Autodesk Inventor part; units mm, degrees
(part 2 of 2)
  spline S324 degree 2 poles (-2.8831, -28.3375) (-2.6289, -28.3375) (-2.4265, -28.3012) (-2.2631, -28.1845) (-2.2009, -28.0807) knots 0 0 0 1 2 3 3 3
  line L148 (-2.2009, -28.0807) -> (-2.1152, -28.0807)
  line L149 (-1.6639, -28.7551) -> (-1.6639, -28.6695)
  spline S325 degree 2 poles (-1.6639, -28.6695) (-1.3578, -28.6644) (-0.8338, -28.392) (-0.3436, -27.7072) (-0.245, -27.2973) knots 0 0 0 1 2 3 3 3
  spline S326 degree 2 poles (-0.245, -27.2973) (-0.6134, -27.5334) (-0.9117, -27.5334) knots 0 0 0 1 1 1
  spline S327 degree 2 poles (-0.9117, -27.5334) (-1.2489, -27.5334) (-1.7262, -27.0172) (-1.7262, -26.5866) knots 0 0 0 1 2 2 2
  spline S328 degree 2 poles (-1.7262, -26.5866) (-1.7262, -26.1716) (-1.4875, -25.8447) knots 0 0 0 1 1 1
  spline S329 degree 2 poles (-1.4875, -25.8447) (-1.1996, -25.4504) (-0.7353, -25.4504) knots 0 0 0 1 1 1
  spline S330 degree 2 poles (-0.7353, -25.4504) (-0.3436, -25.4504) (-0.0634, -25.7747) knots 0 0 0 1 1 1
  spline S331 degree 2 poles (-0.0634, -25.7747) (0.279, -26.1742) (0.279, -26.7604) knots 0 0 0 1 1 1
  spline S332 degree 2 poles (0.279, -26.7604) (0.279, -27.2896) (-0.2424, -28.2052) (-0.7067, -28.5061) knots 0 0 0 1 2 2 2
  spline S333 degree 2 poles (-0.7067, -28.5061) (-1.0855, -28.7551) (-1.529, -28.7551) knots 0 0 0 1 1 1
  line L150 (-1.529, -28.7551) -> (-1.6639, -28.7551)
  spline S334 degree 2 poles (-0.2087, -27.1235) (-0.1672, -26.8201) (-0.1672, -26.6385) knots 0 0 0 1 1 1
  spline S335 degree 2 poles (-0.1672, -26.6385) (-0.1672, -26.4102) (-0.3228, -25.8836) (-0.6056, -25.6035) (-0.7871, -25.6035) knots 0 0 0 1 2 3 3 3
  spline S336 degree 2 poles (-0.7871, -25.6035) (-0.9947, -25.6035) (-1.3085, -25.977) (-1.3085, -26.348) knots 0 0 0 1 2 2 2
  spline S337 degree 2 poles (-1.3085, -26.348) (-1.3085, -26.8408) (-1.101, -27.1184) knots 0 0 0 1 1 1
  spline S338 degree 2 poles (-1.101, -27.1184) (-0.948, -27.3207) (-0.7249, -27.3207) knots 0 0 0 1 1 1
  spline S339 degree 2 poles (-0.7249, -27.3207) (-0.6159, -27.3207) (-0.3202, -27.2169) (-0.2087, -27.1235) knots 0 0 0 1 2 2 2
  line L151 (2.5668, -25.5153) -> (2.3853, -25.9122)
  line L152 (2.3853, -25.9122) -> (1.4307, -25.9122)
  line L153 (1.4307, -25.9122) -> (1.2206, -26.3376)
  spline S340 degree 2 poles (1.2206, -26.3376) (1.8405, -26.4284) (2.2037, -26.7993) knots 0 0 0 1 1 1
  spline S341 degree 2 poles (2.2037, -26.7993) (2.515, -27.1184) (2.515, -27.549) knots 0 0 0 1 1 1
  spline S342 degree 2 poles (2.515, -27.549) (2.515, -27.798) (2.31, -28.226) (2.0014, -28.5243) (1.812, -28.6151) knots 0 0 0 1 2 3 3 3
  spline S343 degree 2 poles (1.812, -28.6151) (1.5422, -28.7448) (1.2595, -28.7448) knots 0 0 0 1 1 1
  spline S344 degree 2 poles (1.2595, -28.7448) (0.9716, -28.7448) (0.7122, -28.5502) (0.7122, -28.4335) knots 0 0 0 1 2 2 2
  spline S345 degree 2 poles (0.7122, -28.4335) (0.7122, -28.3686) (0.8185, -28.2675) (0.9015, -28.2675) knots 0 0 0 1 2 2 2
  spline S346 degree 2 poles (0.9015, -28.2675) (0.9612, -28.2675) (1.0546, -28.3064) (1.1635, -28.3842) knots 0 0 0 1 2 2 2
  spline S347 degree 2 poles (1.1635, -28.3842) (1.3399, -28.5035) (1.5215, -28.5061) knots 0 0 0 1 1 1
  spline S348 degree 2 poles (1.5215, -28.5061) (1.7938, -28.5061) (2.2115, -28.0911) (2.2115, -27.7928) knots 0 0 0 1 2 2 2
  spline S349 degree 2 poles (2.2115, -27.7928) (2.2115, -27.5049) (1.8405, -27.0042) (1.5137, -26.8693) knots 0 0 0 1 2 2 2
  spline S350 degree 2 poles (1.5137, -26.8693) (1.2595, -26.763) (0.8185, -26.7474) knots 0 0 0 1 1 1
  line L154 (0.8185, -26.7474) -> (1.4281, -25.5153)
  line L155 (1.4281, -25.5153) -> (2.5668, -25.5153)
  spline S351 degree 2 poles (3.0571, -27.121) (3.0571, -26.5788) (3.3839, -25.7954) (3.6563, -25.6035) knots 0 0 0 1 2 2 2
  spline S352 degree 2 poles (3.6563, -25.6035) (3.8664, -25.4504) (4.0921, -25.4504) knots 0 0 0 1 1 1
  spline S353 degree 2 poles (4.0921, -25.4504) (4.4578, -25.4504) (4.7484, -25.8214) knots 0 0 0 1 1 1
  spline S354 degree 2 poles (4.7484, -25.8214) (5.1115, -26.2831) (5.1115, -27.0717) knots 0 0 0 1 1 1
  spline S355 degree 2 poles (5.1115, -27.0717) (5.1115, -27.6242) (4.7925, -28.3972) (4.2996, -28.7448) (4.0687, -28.7448) knots 0 0 0 1 2 3 3 3
  spline S356 degree 2 poles (4.0687, -28.7448) (3.6148, -28.7448) (3.3113, -28.2078) knots 0 0 0 1 1 1
  spline S357 degree 2 poles (3.3113, -28.2078) (3.0571, -27.7565) (3.0571, -27.121) knots 0 0 0 1 1 1
  spline S358 degree 2 poles (3.5162, -27.1806) (3.5162, -27.8343) (3.677, -28.2493) knots 0 0 0 1 1 1
  spline S359 degree 2 poles (3.677, -28.2493) (3.8119, -28.5969) (4.0765, -28.5969) knots 0 0 0 1 1 1
  spline S360 degree 2 poles (4.0765, -28.5969) (4.2036, -28.5969) (4.4734, -28.3712) (4.5434, -28.1041) knots 0 0 0 1 2 2 2
  spline S361 degree 2 poles (4.5434, -28.1041) (4.6524, -27.702) (4.6524, -26.9705) knots 0 0 0 1 1 1
  spline S362 degree 2 poles (4.6524, -26.9705) (4.6524, -26.4258) (4.5408, -26.0652) knots 0 0 0 1 1 1
  spline S363 degree 2 poles (4.5408, -26.0652) (4.4552, -25.7954) (4.3229, -25.6839) knots 0 0 0 1 1 1
  spline S364 degree 2 poles (4.3229, -25.6839) (4.227, -25.6061) (4.0895, -25.6061) knots 0 0 0 1 1 1
  spline S365 degree 2 poles (4.0895, -25.6061) (3.9313, -25.6061) (3.8067, -25.7488) knots 0 0 0 1 1 1
  spline S366 degree 2 poles (3.8067, -25.7488) (3.6381, -25.9433) (3.5162, -26.776) (3.5162, -27.1806) knots 0 0 0 1 2 2 2
  spline S367 degree 2 poles (5.4565, -27.121) (5.4565, -26.5788) (5.7833, -25.7954) (6.0557, -25.6035) knots 0 0 0 1 2 2 2
  spline S368 degree 2 poles (6.0557, -25.6035) (6.2658, -25.4504) (6.4915, -25.4504) knots 0 0 0 1 1 1
  spline S369 degree 2 poles (6.4915, -25.4504) (6.8572, -25.4504) (7.1478, -25.8214) knots 0 0 0 1 1 1
  spline S370 degree 2 poles (7.1478, -25.8214) (7.5109, -26.2831) (7.5109, -27.0717) knots 0 0 0 1 1 1
  spline S371 degree 2 poles (7.5109, -27.0717) (7.5109, -27.6242) (7.1919, -28.3972) (6.699, -28.7448) (6.4681, -28.7448) knots 0 0 0 1 2 3 3 3
  spline S372 degree 2 poles (6.4681, -28.7448) (6.0142, -28.7448) (5.7107, -28.2078) knots 0 0 0 1 1 1
  spline S373 degree 2 poles (5.7107, -28.2078) (5.4565, -27.7565) (5.4565, -27.121) knots 0 0 0 1 1 1
  spline S374 degree 2 poles (5.9156, -27.1806) (5.9156, -27.8343) (6.0765, -28.2493) knots 0 0 0 1 1 1
  spline S375 degree 2 poles (6.0765, -28.2493) (6.2113, -28.5969) (6.4759, -28.5969) knots 0 0 0 1 1 1
  spline S376 degree 2 poles (6.4759, -28.5969) (6.603, -28.5969) (6.8728, -28.3712) (6.9428, -28.1041) knots 0 0 0 1 2 2 2
  spline S377 degree 2 poles (6.9428, -28.1041) (7.0518, -27.702) (7.0518, -26.9705) knots 0 0 0 1 1 1
  spline S378 degree 2 poles (7.0518, -26.9705) (7.0518, -26.4258) (6.9402, -26.0652) knots 0 0 0 1 1 1
  spline S379 degree 2 poles (6.9402, -26.0652) (6.8546, -25.7954) (6.7224, -25.6839) knots 0 0 0 1 1 1
  spline S380 degree 2 poles (6.7224, -25.6839) (6.6264, -25.6061) (6.4889, -25.6061) knots 0 0 0 1 1 1
  spline S381 degree 2 poles (6.4889, -25.6061) (6.3307, -25.6061) (6.2062, -25.7488) knots 0 0 0 1 1 1
  spline S382 degree 2 poles (6.2062, -25.7488) (6.0375, -25.9433) (5.9156, -26.776) (5.9156, -27.1806) knots 0 0 0 1 2 2 2
  line L156 (8.2424, -25.8266) -> (9.0154, -25.4504)
  line L157 (9.0154, -25.4504) -> (9.0932, -25.4504)
  line L158 (9.0932, -25.4504) -> (9.0932, -28.13)
  spline S383 degree 2 poles (9.0932, -28.13) (9.0932, -28.3972) (9.1373, -28.5295) (9.2774, -28.5995) (9.4927, -28.6047) knots 0 0 0 1 2 3 3 3
  line L159 (9.4927, -28.6047) -> (9.4927, -28.6903)
  line L160 (9.4927, -28.6903) -> (8.2995, -28.6903)
  line L161 (8.2995, -28.6903) -> (8.2995, -28.6047)
  spline S384 degree 2 poles (8.2995, -28.6047) (8.5252, -28.5995) (8.6548, -28.5321) (8.7067, -28.4179) (8.7067, -28.13) knots 0 0 0 1 2 3 3 3
  line L162 (8.7067, -28.13) -> (8.7067, -26.418)
  spline S385 degree 2 poles (8.7067, -26.418) (8.7067, -26.0704) (8.6834, -25.9718) knots 0 0 0 1 1 1
  spline S386 degree 2 poles (8.6834, -25.9718) (8.6678, -25.8966) (8.5796, -25.8266) (8.52, -25.8266) knots 0 0 0 1 2 2 2
  spline S387 degree 2 poles (8.52, -25.8266) (8.4318, -25.8266) (8.2787, -25.8992) knots 0 0 0 1 1 1
  line L163 (8.2787, -25.8992) -> (8.2424, -25.8266)
  line L164 (-12.1098, -33.1024) -> (-12.3328, -33.712)
  line L165 (-12.3328, -33.712) -> (-14.2057, -33.712)
  line L166 (-14.2057, -33.712) -> (-14.2057, -33.6264)
  spline S388 degree 2 poles (-14.2057, -33.6264) (-13.3782, -32.8716) (-12.7038, -31.917) (-12.7038, -31.5201) knots 0 0 0 1 2 2 2
  spline S389 degree 2 poles (-12.7038, -31.5201) (-12.7038, -31.2192) (-13.0747, -30.8301) (-13.3315, -30.8301) knots 0 0 0 1 2 2 2
  spline S390 degree 2 poles (-13.3315, -30.8301) (-13.5676, -30.8301) (-13.9385, -31.1051) (-14.0293, -31.3697) knots 0 0 0 1 2 2 2
  line L167 (-14.0293, -31.3697) -> (-14.1149, -31.3697)
  spline S391 degree 2 poles (-14.1149, -31.3697) (-14.0552, -30.9365) (-13.5727, -30.4722) (-13.2096, -30.4722) knots 0 0 0 1 2 2 2
  spline S392 degree 2 poles (-13.2096, -30.4722) (-12.8231, -30.4722) (-12.3043, -30.9676) (-12.3043, -31.3048) knots 0 0 0 1 2 2 2
  spline S393 degree 2 poles (-12.3043, -31.3048) (-12.3043, -31.5461) (-12.4158, -31.7873) knots 0 0 0 1 1 1
  spline S394 degree 2 poles (-12.4158, -31.7873) (-12.5896, -32.166) (-12.9787, -32.5914) knots 0 0 0 1 1 1
  spline S395 degree 2 poles (-12.9787, -32.5914) (-13.5624, -33.2269) (-13.7076, -33.3592) knots 0 0 0 1 1 1
  line L168 (-13.7076, -33.3592) -> (-12.8776, -33.3592)
  spline S396 degree 2 poles (-12.8776, -33.3592) (-12.6234, -33.3592) (-12.421, -33.3229) (-12.2576, -33.2062) (-12.1954, -33.1024) knots 0 0 0 1 2 3 3 3
  line L169 (-12.1954, -33.1024) -> (-12.1098, -33.1024)
  spline S397 degree 2 poles (-10.9892, -32.1115) (-11.3653, -31.8029) (-11.5832, -31.4293) (-11.5832, -31.227) knots 0 0 0 1 2 2 2
  spline S398 degree 2 poles (-11.5832, -31.227) (-11.5832, -30.9183) (-11.1059, -30.4722) (-10.709, -30.4722) knots 0 0 0 1 2 2 2
  spline S399 degree 2 poles (-10.709, -30.4722) (-10.3251, -30.4722) (-9.8556, -30.8872) (-9.8556, -31.1544) knots 0 0 0 1 2 2 2
  spline S400 degree 2 poles (-9.8556, -31.1544) (-9.8556, -31.3334) (-10.1098, -31.7017) (-10.5093, -31.9533) knots 0 0 0 1 2 2 2
  spline S401 degree 2 poles (-10.5093, -31.9533) (-10.0968, -32.2698) (-9.9646, -32.4539) knots 0 0 0 1 1 1
  spline S402 degree 2 poles (-9.9646, -32.4539) (-9.7856, -32.6926) (-9.7856, -32.9572) knots 0 0 0 1 1 1
  spline S403 degree 2 poles (-9.7856, -32.9572) (-9.7856, -33.2918) (-10.2966, -33.7665) (-10.7116, -33.7665) knots 0 0 0 1 2 2 2
  spline S404 degree 2 poles (-10.7116, -33.7665) (-11.1656, -33.7665) (-11.4172, -33.4837) knots 0 0 0 1 1 1
  spline S405 degree 2 poles (-11.4172, -33.4837) (-11.6195, -33.2555) (-11.6195, -32.9857) knots 0 0 0 1 1 1
  spline S406 degree 2 poles (-11.6195, -32.9857) (-11.6195, -32.7756) (-11.3368, -32.3632) (-10.9892, -32.1115) knots 0 0 0 1 2 2 2
  spline S407 degree 2 poles (-10.8776, -32.1997) (-11.0748, -32.3632) (-11.2615, -32.7497) (-11.2615, -32.9753) knots 0 0 0 1 2 2 2
  spline S408 degree 2 poles (-11.2615, -32.9753) (-11.2615, -33.2762) (-10.9295, -33.6394) (-10.6753, -33.6394) knots 0 0 0 1 2 2 2
  spline S409 degree 2 poles (-10.6753, -33.6394) (-10.4211, -33.6394) (-10.115, -33.354) (-10.115, -33.1491) knots 0 0 0 1 2 2 2
  spline S410 degree 2 poles (-10.115, -33.1491) (-10.115, -32.9831) (-10.2032, -32.8482) knots 0 0 0 1 1 1
  spline S411 degree 2 poles (-10.2032, -32.8482) (-10.3718, -32.6018) (-10.8776, -32.1997) knots 0 0 0 1 1 1
  spline S412 degree 2 poles (-10.6208, -31.8599) (-10.3381, -31.6083) (-10.1876, -31.3152) (-10.1876, -31.131) knots 0 0 0 1 2 2 2
  spline S413 degree 2 poles (-10.1876, -31.131) (-10.1876, -30.8846) (-10.4652, -30.607) (-10.7038, -30.607) knots 0 0 0 1 2 2 2
  spline S414 degree 2 poles (-10.7038, -30.607) (-10.9425, -30.607) (-11.2434, -30.882) (-11.2434, -31.0688) knots 0 0 0 1 2 2 2
  spline S415 degree 2 poles (-11.2434, -31.0688) (-11.2434, -31.1907) (-11.1189, -31.4319) (-11.0047, -31.5435) knots 0 0 0 1 2 2 2
  line L170 (-11.0047, -31.5435) -> (-10.6208, -31.8599)
  line L171 (-8.735, -30.8613) -> (-8.735, -31.5668)
  line L172 (-8.735, -31.5668) -> (-8.2344, -31.5668)
  line L173 (-8.2344, -31.5668) -> (-8.2344, -31.7302)
  line L174 (-8.2344, -31.7302) -> (-8.735, -31.7302)
  line L175 (-8.735, -31.7302) -> (-8.735, -33.1232)
  spline S416 degree 2 poles (-8.735, -33.1232) (-8.735, -33.3307) (-8.6157, -33.476) (-8.5223, -33.476) knots 0 0 0 1 2 2 2
  spline S417 degree 2 poles (-8.5223, -33.476) (-8.4445, -33.476) (-8.2966, -33.38) (-8.2577, -33.2866) knots 0 0 0 1 2 2 2
  line L176 (-8.2577, -33.2866) -> (-8.1669, -33.2866)
  spline S418 degree 2 poles (-8.1669, -33.2866) (-8.25, -33.5175) (-8.5509, -33.7483) (-8.7091, -33.7483) knots 0 0 0 1 2 2 2
  spline S419 degree 2 poles (-8.7091, -33.7483) (-8.818, -33.7483) (-9.0255, -33.629) (-9.1241, -33.4059) (-9.1241, -33.1751) knots 0 0 0 1 2 3 3 3
  line L177 (-9.1241, -33.1751) -> (-9.1241, -31.7302)
  line L178 (-9.1241, -31.7302) -> (-9.4639, -31.7302)
  line L179 (-9.4639, -31.7302) -> (-9.4639, -31.6524)
  spline S420 degree 2 poles (-9.4639, -31.6524) (-9.3342, -31.6005) (-9.0645, -31.3567) (-8.9581, -31.1881) knots 0 0 0 1 2 2 2
  spline S421 degree 2 poles (-8.9581, -31.1881) (-8.9036, -31.0973) (-8.8077, -30.8613) knots 0 0 0 1 1 1
  line L180 (-8.8077, -30.8613) -> (-8.735, -30.8613)
  line L181 (-7.3965, -30.3814) -> (-7.3965, -31.9507)
  spline S422 degree 2 poles (-7.3965, -31.9507) (-7.1371, -31.6654) (-6.8337, -31.5046) (-6.6806, -31.5046) knots 0 0 0 1 2 2 2
  spline S423 degree 2 poles (-6.6806, -31.5046) (-6.499, -31.5046) (-6.2344, -31.7069) (-6.1722, -31.9222) knots 0 0 0 1 2 2 2
  spline S424 degree 2 poles (-6.1722, -31.9222) (-6.1281, -32.07) (-6.1281, -32.4695) knots 0 0 0 1 1 1
  line L182 (-6.1281, -32.4695) -> (-6.1281, -33.2269)
  spline S425 degree 2 poles (-6.1281, -33.2269) (-6.1281, -33.4293) (-6.0944, -33.5045) knots 0 0 0 1 1 1
  spline S426 degree 2 poles (-6.0944, -33.5045) (-6.071, -33.5616) (-5.9595, -33.6264) (-5.809, -33.6264) knots 0 0 0 1 2 2 2
  line L183 (-5.809, -33.6264) -> (-5.809, -33.712)
  line L184 (-5.809, -33.712) -> (-6.8648, -33.712)
  line L185 (-6.8648, -33.712) -> (-6.8648, -33.6264)
  line L186 (-6.8648, -33.6264) -> (-6.8155, -33.6264)
  spline S427 degree 2 poles (-6.8155, -33.6264) (-6.665, -33.6264) (-6.5483, -33.5356) (-6.525, -33.4474) knots 0 0 0 1 2 2 2
  spline S428 degree 2 poles (-6.525, -33.4474) (-6.5172, -33.4085) (-6.5172, -33.2269) knots 0 0 0 1 1 1
  line L187 (-6.5172, -33.2269) -> (-6.5172, -32.4695)
  spline S429 degree 2 poles (-6.5172, -32.4695) (-6.5172, -32.1167) (-6.5898, -31.8962) (-6.7481, -31.7873) (-6.8622, -31.7873) knots 0 0 0 1 2 3 3 3
  spline S430 degree 2 poles (-6.8622, -31.7873) (-6.9763, -31.7873) (-7.2227, -31.9092) (-7.3965, -32.0934) knots 0 0 0 1 2 2 2
  line L188 (-7.3965, -32.0934) -> (-7.3965, -33.2269)
  spline S431 degree 2 poles (-7.3965, -33.2269) (-7.3965, -33.4474) (-7.3473, -33.5538) (-7.2124, -33.6264) (-7.049, -33.6264) knots 0 0 0 1 2 3 3 3
  line L189 (-7.049, -33.6264) -> (-7.049, -33.712)
  line L190 (-7.049, -33.712) -> (-8.1125, -33.712)
  line L191 (-8.1125, -33.712) -> (-8.1125, -33.6264)
  spline S432 degree 2 poles (-8.1125, -33.6264) (-7.9698, -33.6264) (-7.8894, -33.5823) knots 0 0 0 1 1 1
  spline S433 degree 2 poles (-7.8894, -33.5823) (-7.8427, -33.559) (-7.7856, -33.4267) (-7.7856, -33.2269) knots 0 0 0 1 2 2 2
  line L192 (-7.7856, -33.2269) -> (-7.7856, -31.2841)
  spline S434 degree 2 poles (-7.7856, -31.2841) (-7.7856, -30.9183) (-7.8219, -30.7523) (-7.8946, -30.6926) (-7.9542, -30.6926) knots 0 0 0 1 2 3 3 3
  spline S435 degree 2 poles (-7.9542, -30.6926) (-8.0035, -30.6926) (-8.1125, -30.729) knots 0 0 0 1 1 1
  line L193 (-8.1125, -30.729) -> (-8.1462, -30.6434)
  line L194 (-8.1462, -30.6434) -> (-7.5055, -30.3814)
  line L195 (-7.5055, -30.3814) -> (-7.3965, -30.3814)
  line L196 (-2.3798, -32.6511) -> (-3.6146, -32.6511)
  line L197 (-3.6146, -32.6511) -> (-3.8299, -33.1491)
  spline S436 degree 2 poles (-3.8299, -33.1491) (-3.9103, -33.3359) (-3.9103, -33.4267) knots 0 0 0 1 1 1
  spline S437 degree 2 poles (-3.9103, -33.4267) (-3.9103, -33.4993) (-3.7702, -33.6108) (-3.5419, -33.6264) knots 0 0 0 1 2 2 2
  line L198 (-3.5419, -33.6264) -> (-3.5419, -33.712)
  line L199 (-3.5419, -33.712) -> (-4.5432, -33.712)
  line L200 (-4.5432, -33.712) -> (-4.5432, -33.6264)
  spline S438 degree 2 poles (-4.5432, -33.6264) (-4.3435, -33.5901) (-4.2864, -33.5356) knots 0 0 0 1 1 1
  spline S439 degree 2 poles (-4.2864, -33.5356) (-4.1671, -33.4215) (-4.0218, -33.0765) knots 0 0 0 1 1 1
  line L201 (-4.0218, -33.0765) -> (-2.9012, -30.4644)
  line L202 (-2.9012, -30.4644) -> (-2.8182, -30.4644)
  line L203 (-2.8182, -30.4644) -> (-1.7132, -33.105)
  spline S440 degree 2 poles (-1.7132, -33.105) (-1.5809, -33.4241) (-1.363, -33.6134) (-1.1685, -33.6264) knots 0 0 0 1 2 2 2
  line L204 (-1.1685, -33.6264) -> (-1.1685, -33.712)
  line L205 (-1.1685, -33.712) -> (-2.4213, -33.712)
  line L206 (-2.4213, -33.712) -> (-2.4213, -33.6264)
  spline S441 degree 2 poles (-2.4213, -33.6264) (-2.232, -33.616) (-2.0971, -33.5097) (-2.0971, -33.4319) knots 0 0 0 1 2 2 2
  spline S442 degree 2 poles (-2.0971, -33.4319) (-2.0971, -33.3281) (-2.1905, -33.105) knots 0 0 0 1 1 1
  line L207 (-2.1905, -33.105) -> (-2.3798, -32.6511)
  line L208 (-2.4525, -32.4773) -> (-2.9868, -31.1933)
  line L209 (-2.9868, -31.1933) -> (-3.5419, -32.4773)
  line L210 (-3.5419, -32.4773) -> (-2.4525, -32.4773)
  line L211 (0.9145, -31.5668) -> (0.9145, -32.869)
  spline S443 degree 2 poles (0.9145, -32.869) (0.9145, -33.2373) (0.9508, -33.4033) (1.026, -33.4682) (1.0779, -33.4682) knots 0 0 0 1 2 3 3 3
  spline S444 degree 2 poles (1.0779, -33.4682) (1.1505, -33.4682) (1.2413, -33.4293) knots 0 0 0 1 1 1
  line L212 (1.2413, -33.4293) -> (1.275, -33.5149)
  line L213 (1.275, -33.5149) -> (0.6343, -33.7769)
  line L214 (0.6343, -33.7769) -> (0.528, -33.7769)
  line L215 (0.528, -33.7769) -> (0.528, -33.3229)
  spline S445 degree 2 poles (0.528, -33.3229) (0.2504, -33.6212) (-0.0375, -33.7769) (-0.2009, -33.7769) knots 0 0 0 1 2 2 2
  spline S446 degree 2 poles (-0.2009, -33.7769) (-0.3799, -33.7769) (-0.6445, -33.5693) (-0.7482, -33.2399) (-0.7482, -32.9416) knots 0 0 0 1 2 3 3 3
  line L216 (-0.7482, -32.9416) -> (-0.7482, -31.9844)
  spline S447 degree 2 poles (-0.7482, -31.9844) (-0.7482, -31.8314) (-0.8131, -31.7147) (-0.9428, -31.6498) (-1.1114, -31.6524) knots 0 0 0 1 2 3 3 3
  line L217 (-1.1114, -31.6524) -> (-1.1114, -31.5668)
  line L218 (-1.1114, -31.5668) -> (-0.3591, -31.5668)
  line L219 (-0.3591, -31.5668) -> (-0.3591, -33.0013)
  spline S448 degree 2 poles (-0.3591, -33.0013) (-0.3591, -33.3022) (-0.1516, -33.4889) (-0.0038, -33.4889) knots 0 0 0 1 2 2 2
  spline S449 degree 2 poles (-0.0038, -33.4889) (0.0974, -33.4889) (0.3516, -33.3618) (0.528, -33.1854) knots 0 0 0 1 2 2 2
  line L220 (0.528, -33.1854) -> (0.528, -31.9689)
  spline S450 degree 2 poles (0.528, -31.9689) (0.528, -31.7873) (0.3931, -31.6576) (0.1804, -31.6524) knots 0 0 0 1 2 2 2
  line L221 (0.1804, -31.6524) -> (0.1804, -31.5668)
  line L222 (0.1804, -31.5668) -> (0.9145, -31.5668)
  spline S451 degree 2 poles (2.0065, -32.9286) (1.8094, -32.8327) (1.5993, -32.4903) (1.5993, -32.2801) knots 0 0 0 1 2 2 2
  spline S452 degree 2 poles (1.5993, -32.2801) (1.5993, -31.9637) (2.0792, -31.5046) (2.4553, -31.5046) knots 0 0 0 1 2 2 2
  spline S453 degree 2 poles (2.4553, -31.5046) (2.7614, -31.5046) (2.9871, -31.655) knots 0 0 0 1 1 1
  line L223 (2.9871, -31.655) -> (3.441, -31.655)
  spline S454 degree 2 poles (3.441, -31.655) (3.5422, -31.655) (3.5759, -31.6654) (3.5837, -31.6809) knots 0 0 0 1 2 2 2
  spline S455 degree 2 poles (3.5837, -31.6809) (3.5966, -31.7017) (3.5966, -31.7562) knots 0 0 0 1 1 1
  spline S456 degree 2 poles (3.5966, -31.7562) (3.5966, -31.8158) (3.5837, -31.8392) knots 0 0 0 1 1 1
  spline S457 degree 2 poles (3.5837, -31.8392) (3.5785, -31.8521) (3.5422, -31.8651) (3.441, -31.8651) knots 0 0 0 1 2 2 2
  line L224 (3.441, -31.8651) -> (3.1609, -31.8651)
  spline S458 degree 2 poles (3.1609, -31.8651) (3.2931, -32.0337) (3.2931, -32.2957) knots 0 0 0 1 1 1
  spline S459 degree 2 poles (3.2931, -32.2957) (3.2931, -32.5966) (2.834, -33.022) (2.4475, -33.022) knots 0 0 0 1 2 2 2
  spline S460 degree 2 poles (2.4475, -33.022) (2.2893, -33.022) (2.1207, -32.9753) knots 0 0 0 1 1 1
  spline S461 degree 2 poles (2.1207, -32.9753) (2.0195, -33.0635) (1.9469, -33.1958) (1.9469, -33.2425) knots 0 0 0 1 2 2 2
  spline S462 degree 2 poles (1.9469, -33.2425) (1.9469, -33.284) (2.0247, -33.3592) (2.1362, -33.3748) knots 0 0 0 1 2 2 2
  spline S463 degree 2 poles (2.1362, -33.3748) (2.2011, -33.3852) (2.4657, -33.3904) knots 0 0 0 1 1 1
  spline S464 degree 2 poles (2.4657, -33.3904) (2.9481, -33.4033) (3.0908, -33.4241) knots 0 0 0 1 1 1
  spline S465 degree 2 poles (3.0908, -33.4241) (3.3087, -33.4552) (3.5681, -33.7172) (3.5681, -33.9066) knots 0 0 0 1 2 2 2
  spline S466 degree 2 poles (3.5681, -33.9066) (3.5681, -34.1711) (3.3191, -34.402) knots 0 0 0 1 1 1
  spline S467 degree 2 poles (3.3191, -34.402) (2.9533, -34.7444) (2.3645, -34.7444) knots 0 0 0 1 1 1
  spline S468 degree 2 poles (2.3645, -34.7444) (1.9132, -34.7444) (1.6019, -34.5421) knots 0 0 0 1 1 1
  spline S469 degree 2 poles (1.6019, -34.5421) (1.4255, -34.4253) (1.4255, -34.2982) knots 0 0 0 1 1 1
  spline S470 degree 2 poles (1.4255, -34.2982) (1.4255, -34.2412) (1.4514, -34.1867) knots 0 0 0 1 1 1
  spline S471 degree 2 poles (1.4514, -34.1867) (1.4903, -34.0985) (1.6149, -33.9455) knots 0 0 0 1 1 1
  spline S472 degree 2 poles (1.6149, -33.9455) (1.633, -33.9247) (1.8535, -33.6939) knots 0 0 0 1 1 1
  spline S473 degree 2 poles (1.8535, -33.6939) (1.7342, -33.6212) (1.633, -33.5045) (1.633, -33.4319) knots 0 0 0 1 2 2 2
  spline S474 degree 2 poles (1.633, -33.4319) (1.633, -33.3515) (1.7653, -33.131) (2.0065, -32.9286) knots 0 0 0 1 2 2 2
  spline S475 degree 2 poles (1.9832, -33.712) (1.8717, -33.8313) (1.7601, -34.0363) (1.7601, -34.1219) knots 0 0 0 1 2 2 2
  spline S476 degree 2 poles (1.7601, -34.1219) (1.7601, -34.2334) (1.895, -34.3164) knots 0 0 0 1 1 1
  spline S477 degree 2 poles (1.895, -34.3164) (2.1311, -34.4617) (2.5746, -34.4617) knots 0 0 0 1 1 1
  spline S478 degree 2 poles (2.5746, -34.4617) (2.9948, -34.4617) (3.3969, -34.166) (3.3969, -33.9999) knots 0 0 0 1 2 2 2
  spline S479 degree 2 poles (3.3969, -33.9999) (3.3969, -33.878) (3.2776, -33.8261) knots 0 0 0 1 1 1
  spline S480 degree 2 poles (3.2776, -33.8261) (3.1557, -33.7769) (2.7951, -33.7665) knots 0 0 0 1 1 1
  spline S481 degree 2 poles (2.7951, -33.7665) (2.2659, -33.7535) (1.9832, -33.712) knots 0 0 0 1 1 1
  spline S482 degree 2 poles (2.4138, -31.6161) (2.24, -31.6161) (2.0065, -31.8911) (2.0065, -32.1764) knots 0 0 0 1 2 2 2
  spline S483 degree 2 poles (2.0065, -32.1764) (2.0065, -32.5473) (2.1648, -32.7497) knots 0 0 0 1 1 1
  spline S484 degree 2 poles (2.1648, -32.7497) (2.2867, -32.9053) (2.476, -32.9053) knots 0 0 0 1 1 1
  spline S485 degree 2 poles (2.476, -32.9053) (2.6524, -32.9053) (2.8833, -32.6381) (2.8833, -32.3528) knots 0 0 0 1 2 2 2
  spline S486 degree 2 poles (2.8833, -32.3528) (2.8833, -31.9818) (2.7225, -31.7717) knots 0 0 0 1 1 1
  spline S487 degree 2 poles (2.7225, -31.7717) (2.6032, -31.6161) (2.4138, -31.6161) knots 0 0 0 1 1 1
  line L225 (7.0803, -33.1024) -> (6.8572, -33.712)
  line L226 (6.8572, -33.712) -> (4.9844, -33.712)
  line L227 (4.9844, -33.712) -> (4.9844, -33.6264)
  spline S488 degree 2 poles (4.9844, -33.6264) (5.8119, -32.8716) (6.4863, -31.917) (6.4863, -31.5201) knots 0 0 0 1 2 2 2
  spline S489 degree 2 poles (6.4863, -31.5201) (6.4863, -31.2192) (6.1154, -30.8301) (5.8586, -30.8301) knots 0 0 0 1 2 2 2
  spline S490 degree 2 poles (5.8586, -30.8301) (5.6225, -30.8301) (5.2516, -31.1051) (5.1608, -31.3697) knots 0 0 0 1 2 2 2
  line L228 (5.1608, -31.3697) -> (5.0752, -31.3697)
  spline S491 degree 2 poles (5.0752, -31.3697) (5.1349, -30.9365) (5.6173, -30.4722) (5.9805, -30.4722) knots 0 0 0 1 2 2 2
  spline S492 degree 2 poles (5.9805, -30.4722) (6.367, -30.4722) (6.8858, -30.9676) (6.8858, -31.3048) knots 0 0 0 1 2 2 2
  spline S493 degree 2 poles (6.8858, -31.3048) (6.8858, -31.5461) (6.7742, -31.7873) knots 0 0 0 1 1 1
  spline S494 degree 2 poles (6.7742, -31.7873) (6.6004, -32.166) (6.2113, -32.5914) knots 0 0 0 1 1 1
  spline S495 degree 2 poles (6.2113, -32.5914) (5.6277, -33.2269) (5.4824, -33.3592) knots 0 0 0 1 1 1
  line L229 (5.4824, -33.3592) -> (6.3125, -33.3592)
  spline S496 degree 2 poles (6.3125, -33.3592) (6.5667, -33.3592) (6.769, -33.3229) (6.9325, -33.2062) (6.9947, -33.1024) knots 0 0 0 1 2 3 3 3
  line L230 (6.9947, -33.1024) -> (7.0803, -33.1024)
  spline S497 degree 2 poles (7.4538, -32.1427) (7.4538, -31.6005) (7.7807, -30.8172) (8.0531, -30.6252) knots 0 0 0 1 2 2 2
  spline S498 degree 2 poles (8.0531, -30.6252) (8.2632, -30.4722) (8.4888, -30.4722) knots 0 0 0 1 1 1
  spline S499 degree 2 poles (8.4888, -30.4722) (8.8546, -30.4722) (9.1451, -30.8431) knots 0 0 0 1 1 1
  spline S500 degree 2 poles (9.1451, -30.8431) (9.5083, -31.3048) (9.5083, -32.0934) knots 0 0 0 1 1 1
  spline S501 degree 2 poles (9.5083, -32.0934) (9.5083, -32.6459) (9.1892, -33.4189) (8.6964, -33.7665) (8.4655, -33.7665) knots 0 0 0 1 2 3 3 3
  spline S502 degree 2 poles (8.4655, -33.7665) (8.0115, -33.7665) (7.7081, -33.2295) knots 0 0 0 1 1 1
  spline S503 degree 2 poles (7.7081, -33.2295) (7.4538, -32.7782) (7.4538, -32.1427) knots 0 0 0 1 1 1
  spline S504 degree 2 poles (7.913, -32.2023) (7.913, -32.856) (8.0738, -33.271) knots 0 0 0 1 1 1
  spline S505 degree 2 poles (8.0738, -33.271) (8.2087, -33.6186) (8.4733, -33.6186) knots 0 0 0 1 1 1
  spline S506 degree 2 poles (8.4733, -33.6186) (8.6004, -33.6186) (8.8701, -33.393) (8.9402, -33.1258) knots 0 0 0 1 2 2 2
  spline S507 degree 2 poles (8.9402, -33.1258) (9.0491, -32.7237) (9.0491, -31.9922) knots 0 0 0 1 1 1
  spline S508 degree 2 poles (9.0491, -31.9922) (9.0491, -31.4475) (8.9376, -31.0869) knots 0 0 0 1 1 1
  spline S509 degree 2 poles (8.9376, -31.0869) (8.852, -30.8172) (8.7197, -30.7056) knots 0 0 0 1 1 1
  spline S510 degree 2 poles (8.7197, -30.7056) (8.6237, -30.6278) (8.4862, -30.6278) knots 0 0 0 1 1 1
  spline S511 degree 2 poles (8.4862, -30.6278) (8.328, -30.6278) (8.2035, -30.7705) knots 0 0 0 1 1 1
  spline S512 degree 2 poles (8.2035, -30.7705) (8.0349, -30.965) (7.913, -31.7977) (7.913, -32.2023) knots 0 0 0 1 2 2 2
  line L231 (11.8791, -33.1024) -> (11.6561, -33.712)
  line L232 (11.6561, -33.712) -> (9.7832, -33.712)
  line L233 (9.7832, -33.712) -> (9.7832, -33.6264)
  spline S513 degree 2 poles (9.7832, -33.6264) (10.6107, -32.8716) (11.2851, -31.917) (11.2851, -31.5201) knots 0 0 0 1 2 2 2
  spline S514 degree 2 poles (11.2851, -31.5201) (11.2851, -31.2192) (10.9142, -30.8301) (10.6574, -30.8301) knots 0 0 0 1 2 2 2
  spline S515 degree 2 poles (10.6574, -30.8301) (10.4213, -30.8301) (10.0504, -31.1051) (9.9596, -31.3697) knots 0 0 0 1 2 2 2
  line L234 (9.9596, -31.3697) -> (9.874, -31.3697)
  spline S516 degree 2 poles (9.874, -31.3697) (9.9337, -30.9365) (10.4161, -30.4722) (10.7793, -30.4722) knots 0 0 0 1 2 2 2
  spline S517 degree 2 poles (10.7793, -30.4722) (11.1658, -30.4722) (11.6846, -30.9676) (11.6846, -31.3048) knots 0 0 0 1 2 2 2
  spline S518 degree 2 poles (11.6846, -31.3048) (11.6846, -31.5461) (11.573, -31.7873) knots 0 0 0 1 1 1
  spline S519 degree 2 poles (11.573, -31.7873) (11.3993, -32.166) (11.0102, -32.5914) knots 0 0 0 1 1 1
  spline S520 degree 2 poles (11.0102, -32.5914) (10.4265, -33.2269) (10.2813, -33.3592) knots 0 0 0 1 1 1
  line L235 (10.2813, -33.3592) -> (11.1113, -33.3592)
  spline S521 degree 2 poles (11.1113, -33.3592) (11.3655, -33.3592) (11.5679, -33.3229) (11.7313, -33.2062) (11.7935, -33.1024) knots 0 0 0 1 2 3 3 3
  line L236 (11.7935, -33.1024) -> (11.8791, -33.1024)
  line L237 (14.1618, -30.537) -> (13.9802, -30.9339)
  line L238 (13.9802, -30.9339) -> (13.0257, -30.9339)
  line L239 (13.0257, -30.9339) -> (12.8156, -31.3593)
  spline S522 degree 2 poles (12.8156, -31.3593) (13.4355, -31.4501) (13.7987, -31.821) knots 0 0 0 1 1 1
  spline S523 degree 2 poles (13.7987, -31.821) (14.1099, -32.1401) (14.1099, -32.5707) knots 0 0 0 1 1 1
  spline S524 degree 2 poles (14.1099, -32.5707) (14.1099, -32.8197) (13.905, -33.2477) (13.5963, -33.546) (13.407, -33.6368) knots 0 0 0 1 2 3 3 3
  spline S525 degree 2 poles (13.407, -33.6368) (13.1372, -33.7665) (12.8545, -33.7665) knots 0 0 0 1 1 1
  spline S526 degree 2 poles (12.8545, -33.7665) (12.5665, -33.7665) (12.3071, -33.5719) (12.3071, -33.4552) knots 0 0 0 1 2 2 2
  spline S527 degree 2 poles (12.3071, -33.4552) (12.3071, -33.3904) (12.4135, -33.2892) (12.4965, -33.2892) knots 0 0 0 1 2 2 2
  spline S528 degree 2 poles (12.4965, -33.2892) (12.5562, -33.2892) (12.6495, -33.3281) (12.7585, -33.4059) knots 0 0 0 1 2 2 2
  spline S529 degree 2 poles (12.7585, -33.4059) (12.9349, -33.5252) (13.1164, -33.5278) knots 0 0 0 1 1 1
  spline S530 degree 2 poles (13.1164, -33.5278) (13.3888, -33.5278) (13.8064, -33.1128) (13.8064, -32.8145) knots 0 0 0 1 2 2 2
  spline S531 degree 2 poles (13.8064, -32.8145) (13.8064, -32.5266) (13.4355, -32.0259) (13.1087, -31.8911) knots 0 0 0 1 2 2 2
  spline S532 degree 2 poles (13.1087, -31.8911) (12.8545, -31.7847) (12.4135, -31.7691) knots 0 0 0 1 1 1
  line L240 (12.4135, -31.7691) -> (13.0231, -30.537)
  line L241 (13.0231, -30.537) -> (14.1618, -30.537)
  point P0 (25.4, -19.05)
  dimension "d0" = 53.086
  dimension "d1" = 50.8
  constraints: 4 other
emboss "Emboss1" sketch "Sketch8" operation cut depth 2 direction (0, 0, 1)
body "Solid1"
